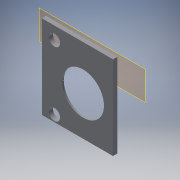
# Autodesk Inventor part: 00_PDMS_chamber_fluidic_v0
Saved by Autodesk Inventor 2019.4 (Build 234330000, 330)
## iProperties
Created: 2021-04-19
Part Number: 00_PDMS_chamber_fluidic_v0
Material: Generic
Document SubType Name: Modeling
Designer: diederichbenedict
Density: 1 g/cm^3
Appearance: White
Author: diederichbenedict
Autodesk Inventor part; units mm, degrees
ref_plane "YZ Plane" through (0, 0, 0) normal (1, 0, 0) x (0, 1, 0)
ref_plane "XZ Plane" through (0, 0, 0) normal (0, 1, 0) x (-1, 0, 0)
ref_plane "Work Plane1" through (-1, 1, 0) normal (0, 0, 1) x (1, 0, 0)
sketch "Sketch1" plane through (-1, 1, 0) normal (0, 0, 1) x (1, 0, 0)
  circle A0 centre (-8, 7.7) radius 1.35 projected
  circle A1 centre (-8, -7.7) radius 1.35 projected
  circle A2 centre (-1.159, 0.036) radius 6 construction
  line L0 (-12, 11.7) -> (6, 11.7)
  line L1 (6, 11.7) -> (6, -11.7)
  line L2 (6, -11.7) -> (-12, -11.7)
  line L3 (-12, -11.7) -> (-12, 11.7)
  point P0 (1, -1)
  dimension "d0" = 18
  dimension "d2" = 4
  dimension "d3" = 4
  dimension "d12" = 4
  constraints: 8 end point, 2 parallel, 1 horizontal, 1 perpendicular
  measures "d0" distance of L1.end L2.end
  measures "d2" distance from line of L0 A0.centre
  measures "d3" distance from line of L3 A0.centre
  measures "d12" distance from line of L2 A1.centre
extrude "Extrusion1" add sketch "Sketch1" along normal blind 1
sketch "Sketch2" plane through (-1, 1, 1) normal (0, 0, 1) x (1, 0, 0)
  circle A0 centre (-1.159, 0.036) radius 6 projected
  circle A1 centre (-1.159, 0.036) radius 5
  point P0 (1, -1)
  dimension "d6" = 10
  constraints: 1 centre point, 1 coincident
  measures "d6" diameter of A1
extrude "Extrusion2" cut sketch "Sketch2" against normal through all contours A1
sketch "Sketch3" plane through (-1, 1, 0) normal (0, 0, -1) x (-1, 0, 0)
  circle A0 centre (1.159, 0.036) radius 5 projected
  circle A1 centre (1.159, 0.036) radius 6.25
  point P0 (-1, -1)
  dimension "d9" = 12.5
  constraints: 1 centre point, 1 coincident
  measures "d9" diameter of A1
ref_plane "Work Plane2" through (-8.159, -4.964, 0.6) normal (0, 0, -1) x (0, 1, 0)
extrude "Extrusion3" cut sketch "Sketch3" against normal up to surface (0.6 mm away)
sketch "Sketch4" plane through (-1, 1, 0) normal (0, 0, -1) x (-1, 0, 0)
  circle A0 centre (8, 7.7) radius 1.35 projected
  circle A1 centre (8, -7.7) radius 1.35 projected
  circle A2 centre (1.159, 0.036) radius 6.25 projected
  line L0 (8, 9.05) -> (0.0063, 9.05)
  line L1 (0.0063, 9.05) -> (0.0063, 6.35)
  line L2 (0.0063, 6.35) -> (8, 6.35)
  line L3 (8, 6.35) -> (8, 9.05)
  line L4 (8, -6.35) -> (0.0063, -6.35)
  line L5 (0.0063, -6.35) -> (0.0063, -9.05)
  line L6 (0.0063, -9.05) -> (8, -9.05)
  line L7 (8, -9.05) -> (8, -6.35)
  line L8 (0.0063, -6.35) -> (0.0063, -6.1068)
  line L9 (3.5216, -6.35) -> (3.5216, -5.7502)
  circle A3 centre (1.159, 0.036) radius 6.25 projected
  line L10 (3.9246, 6.35) -> (3.9246, 5.6409)
  line L11 (0.0063, 6.35) -> (0.0063, 6.1788)
  point P0 (-1, -1)
  constraints: 24 end point, 6 parallel, 5 point on line, 3 point on circle, 2 horizontal, 2 perpendicular, 2 vertical alignment, 1 vertical, 4 other
extrude "Extrusion4" cut sketch "Sketch4" against normal blind 0.5 contours L3 A0 | A0 L2 L1 L0 | L10 A2 L11 L2 | A2 | A2 L9 L4 L8 | L4 A1 L6 L5 | L7 A1 picked at (7.3128, 7.4828) picked at (7.2624, -7.8211)
sketch "Sketch5" plane through (-1, 1, 1) normal (0, 0, 1) x (1, 0, 0)
  circle A0 centre (-8, 7.7) radius 0.5 projected
  circle A1 centre (-8, 7.7) radius 1.35 projected
  circle A2 centre (-8, -7.7) radius 0.5 projected
  circle A3 centre (-8, -7.7) radius 1.35 projected
  arc A4 (-8, 9.05) -> (-8, 6.35) centre (-8, 7.7) ccw projected
  circle A5 centre (-8, 7.7) radius 2.5
  circle A6 centre (-8, -7.7) radius 2.5
  point P0 (1, -1)
  dimension "d15" = 5
  dimension "d16" = 5
  constraints: 2 centre point, 2 coincident
  measures "d15" diameter of A5
  measures "d16" diameter of A6
extrude "Extrusion5" add sketch "Sketch5" along normal blind 2 contours A5 | A6
body "Solid1"
